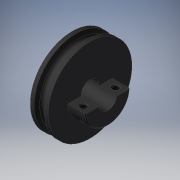
# Autodesk Inventor part: MBRAC45-2-10p1
Saved by Autodesk Inventor 2019 (Build 230136000, 136)
## iProperties
Created: 2024-03-05
Part Number: MBRAC45-2-10p1
Material: Generic
Catalog Web Link: www.cadenas.de
Description: MBRC, MBRAC-p1-Pulleys for Round Belts - Clamping
Vendor: MISUMI
Document SubType Name: Modeling
Designer: psAdmin
Manufacturer: MISUMI
Mass: 16.7743 g
Surface Area: 62.3936 cm^2
Volume: 16.7743 cm^3
Density: 1 g/cm^3
Appearance: PSOLRGB-175-175-175
Category: PARTsolutions
Company: MISUMI
Title: MBRAC45-2-10
Author: Cadenas PARTsolutions
Comments: Pulleys for Round Belts - Clamping
PSOL_IDENT_0: {$CADENAS_DATA/23d-libs/misumi/metric/52_belts_pulleys/mbrc_part1.prj},195 {VTYP=3D},{NB=MBRAC45-2-1
PSOL_IDENT_1: 0p1},{LINA=MBRAC45-2-10},{NN=MBRC, MBRAC-p1},{DATE=01.02.2024 02:39:29},{GEOMDATE=19.01.2024 07:25:3
PSOL_IDENT_2: 2},{VERSION=},{LINEID=30},{WBVAR=MAT,PD,DDS,ALT1},{WBNUMERIC=PD,DDS}  {NB=MBRAC45-2-10p1},{LINA=MBRA
PSOL_IDENT_3: C45-2-10},{KT=DUMMY},{PN=MBRAC45-2-10},{TYPE=MBRAC},{MAT=2},{ST=Clear Anodizing},{AC=Hexagon Socket
PSOL_IDENT_4: Head Cap Screw (2Pcs.) Stainless Steel},{PD=45},{PD0=23,28,30,40,45,48,60,80},{R=2.0},{DDS=10.00},{D
PSOL_IDENT_5: S0=5,6,6.35,8,10,11,12},{D=25},{D1=47},{D2=41},{L=20},{T=10},{LL=4.5},{X=9.0},{Y=4.5},{M=M4},{MM=4.0
PSOL_IDENT_6: 00},{MMMIN=3.242},{CBD=4},{DD1=8.0},{DD2=3.5},{ALT1=},{ALT1ALG='','w/o DC (Outer Diameter Cut)','-DC'
PSOL_IDENT_7: ,'with DC (Outer Diameter Cut)'},{DC=0.0}
NB: MBRAC45-2-10p1
NN: MBRC, MBRAC-p1
NT: Pulleys for Round Belts - Clamping
NBSYN: $PN.p1
LINA: MBRAC45-2-10
CATALOG: Misumi
PN: MBRAC45-2-10
TYPE: MBRAC
MAT: 5052 Aluminum
ST: Clear Anodizing
AC: Hexagon Socket Head Cap Screw (2Pcs.) Stainless Steel
PD: 45
R: 2
DDS: 10
D: 25
D1: 47
D2: 41
L: 20
T: 10
LL: 4.5
X: 9
Y: 4.5
M: M4
CBD: 4
ALT1: w/o DC (Outer Diameter Cut)
DC: 0
SUPPLIER: MISUMI
ARTICLENO: MBRAC45-2-10p1
BOMINFO: MBRAC45-2-10
CREATOR: CADENAS GmbH
Autodesk Inventor part; units mm, degrees
sketch "Sketch_1" plane through (0, 0, 0) normal (0, 0, 1) x (1, 0, 0)
  line L0 (5, 0) -> (-5, 0)
  line L1 (-5, 0) -> (-5, 23.5)
  line L2 (-5, 23.5) -> (-2.8868, 23.5)
  line L3 (-2.8868, 23.5) -> (-1.7321, 21.5)
  arc A0 (-1.7321, 21.5) -> (1.7321, 21.5) centre (0, 22.5) ccw
  line L4 (1.7321, 21.5) -> (2.8868, 23.5)
  line L5 (2.8868, 23.5) -> (5, 23.5)
  line L6 (5, 23.5) -> (5, 0)
  line L7 (5, 0) -> (-5, 0)
  constraints: 16 end point, 2 point on circle, 1 centre point
revolve "Revolution1" add sketch "Sketch_1" angle 360 about axis through (5, 0, 0) along (1, 0, 0)
sketch "Sketch_2" plane through (0, 0, 0) normal (0, 0, 1) x (1, 0, 0)
  line L0 (5, 0) -> (15, 0)
  line L1 (15, 0) -> (15, -12)
  line L2 (15, -12) -> (14.5, -12.5)
  line L3 (14.5, -12.5) -> (5, -12.5)
  line L4 (5, -12.5) -> (5, 0)
  line L5 (5, 0) -> (15, 0)
  constraints: 12 end point
revolve "Revolution2" add sketch "Sketch_2" angle 180 mid plane about axis through (5, 0, 0) along (1, 0, 0)
sketch "Sketch_3" plane through (0, 0, 0) normal (0, 0, 1) x (1, 0, 0)
  line L0 (5, -0.5) -> (15, -0.5)
  line L1 (15, -0.5) -> (15, 0)
  line L2 (15, 0) -> (5, 0)
  line L3 (5, 0) -> (5, -0.5)
  constraints: 8 end point
extrude "Extrusion1" cut sketch "Sketch_3" along normal mid plane 50
sketch "Sketch_4" plane through (0, 0, 0) normal (0, 0, 1) x (1, 0, 0)
  line L0 (15, 0) -> (-5, 0)
  line L1 (-5, 0) -> (-5, 5)
  line L2 (-5, 5) -> (15, 5)
  line L3 (15, 5) -> (15, 0)
  line L4 (15, 0) -> (-5, 0)
  constraints: 10 end point
revolve "Revolution3" cut sketch "Sketch_4" angle 360 about axis through (15, 0, 0) along (1, 0, 0)
sketch "Sketch_5" plane through (0, 0, 9) normal (0, 0, 1) x (1, 0, 0)
  line L0 (10.5, -12.5) -> (10.5, -0.5)
  line L1 (10.5, -0.5) -> (12.5, -0.5)
  line L2 (12.5, -0.5) -> (12.121, -0.879)
  line L3 (12.121, -0.879) -> (12.121, -12.121)
  line L4 (12.121, -12.121) -> (12.5, -12.5)
  line L5 (12.5, -12.5) -> (10.5, -12.5)
  line L6 (10.5, -12.5) -> (10.5, -0.5)
  constraints: 14 end point
revolve "Revolution4" cut sketch "Sketch_5" angle 360 about axis through (10.5, -12.5, 9) along (0, -1, 0)
thread "Thread1" size "M4x0.7" class "6H" standard "ISO Metric profile" length 11.242
sketch "Sketch_6" plane through (0, 0, -9) normal (0, 0, 1) x (1, 0, 0)
  line L0 (10.5, -12.5) -> (10.5, -0.5)
  line L1 (10.5, -0.5) -> (12.5, -0.5)
  line L2 (12.5, -0.5) -> (12.121, -0.879)
  line L3 (12.121, -0.879) -> (12.121, -12.121)
  line L4 (12.121, -12.121) -> (12.5, -12.5)
  line L5 (12.5, -12.5) -> (10.5, -12.5)
  line L6 (10.5, -12.5) -> (10.5, -0.5)
  constraints: 14 end point
revolve "Revolution5" cut sketch "Sketch_6" angle 360 about axis through (10.5, -12.5, -9) along (0, -1, 0)
thread "Thread2" size "M4x0.7" class "6H" standard "ISO Metric profile" length 11.242
ref_plane "part1_to_part2_XY" through (5, 0, 0) normal (1, 0, 0) x (0, 0, -1)
ref_plane "part1_to_part2_YZ" through (5, 0, 0) normal (0, 0, -1) x (0, 1, 0)
ref_plane "part1_to_part2_ZX" through (5, 0, 0) normal (0, 1, 0) x (1, 0, 0)
body "Solid1"
